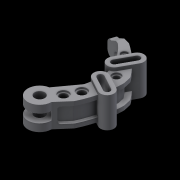
# Autodesk Inventor part: new clamp
Saved by Autodesk Inventor 2015 (Build 190159000, 159)
## iProperties
Created: 2014-10-18
Part Number: new clamp
Material: Generic
Document SubType Name: Modeling
Designer: Inventor
Mass: 7.61279 g
Surface Area: 66.4812 cm^2
Volume: 7.61279 cm^3
Density: 1 g/cm^3
Appearance: Default
RuleStatus: InUse
BeforeDocSave0: UpdateBoundingBox
CX: 35.89 mm
CY: 63.14 mm
CZ: 18.00 mm
Author: Inventor
Autodesk Inventor part; units mm, degrees
ref_plane "YZ Plane" through (0, 0, 0) normal (1, 0, 0) x (0, 1, 0)
ref_plane "XZ Plane" through (0, 0, 0) normal (0, 1, 0) x (-1, 0, 0)
ref_plane "XY Plane" through (0, 0, 0) normal (0, 0, 1) x (1, 0, 0)
sketch "Base" plane through (0, 0, 0) normal (0, 0, 1) x (1, 0, 0)
  circle A0 centre (0, 0) radius 26 construction
  line L0 (17.6916, -25.456) -> (27.5664, -11.8645) construction
  line L1 (27.5664, -11.8645) -> (28.9894, 8.4858) construction
  line L2 (28.9894, 8.4858) -> (16.9443, 25.688) construction
  line L3 (16.9443, 25.688) -> (5.3532, 28.7938) construction
  arc A1 (30.9898, -18.2111) -> (36.4924, 5.7494) centre (-19.9066, 6.0896) ccw
  line L4 (24.6916, -25.4563) -> (30.9898, -18.2111)
  arc A2 (35.4682, 10.4389) -> (17.4626, 27.6222) centre (-24.5964, -34.4748) ccw
  line L5 (35.4682, 10.4389) -> (36.4924, 5.7494)
  line L6 (17.4626, 27.6222) -> (5.8715, 30.728)
  line L7 (5.8715, 30.728) -> (4.9656, 27.3473)
  arc A3 (25.6196, 7.5403) -> (14.0958, 24.3807) centre (-10.6938, -4.9457) ccw
  line L8 (4.9656, 27.3473) -> (14.0958, 24.3807)
  circle A4 centre (17.6916, -25.456) radius 7
  line L9 (25.1124, -6.7357) -> (16.5261, -18.5537)
  circle A5 centre (29.4754, 20.4271) radius 1.75 construction
  line L10 (29.4754, 20.4271) -> (24.6884, 11.6473) construction
  circle A6 centre (24.6884, 11.6473) radius 1.75 construction
  circle A7 centre (29.4754, 20.4271) radius 4
  circle A8 centre (24.6884, 11.6473) radius 4
  circle A9 centre (28.0765, 0.1355) radius 1.75 construction
  line L11 (28.0765, 0.1355) -> (36.8564, -4.6514) construction
  circle A10 centre (36.8564, -4.6514) radius 1.75 construction
  circle A11 centre (36.8564, -4.6514) radius 4
  circle A12 centre (28.0765, 0.1355) radius 4
  line L12 (21.1765, 13.562) -> (25.9634, 22.3419)
  line L13 (28.2004, 9.7325) -> (32.9873, 18.5123)
  line L14 (29.9913, 3.6474) -> (38.7711, -1.1395)
  line L15 (26.1618, -3.3764) -> (34.9416, -8.1633)
  arc A13 (25.1124, -6.7357) -> (25.6196, 7.5403) centre (-5.602, 1.5026) ccw
  line L16 (0, 0) -> (26.0993, 7.6814) construction
  line L17 (16.9443, 25.688) -> (17.4626, 27.6222) construction
  line L18 (0, -47.5154) -> (0, 43.7686) construction
  line L19 (14.0958, 24.3807) -> (14.6134, 26.3126) construction
  line L20 (23.0874, 16.9148) -> (27.1832, 19.7827) construction
  line L21 (34.2322, -9.7203) -> (27.748, -9.2669) construction
  line L22 (24.6884, 11.6473) -> (28.0765, 0.1355) construction
  line L23 (-39.3713, 0) -> (54.2276, 0) construction
  line L24 (26.0993, 7.6814) -> (35.4682, 10.4389) construction
  dimension "d299" = 52
  dimension "d94" = 14
  dimension "d110" = 20.4
  dimension "d111" = 141
  dimension "d112" = 21
  dimension "d122" = 3.5
  dimension "d124" = 8
  dimension "d137" = 16.8
  dimension "d138" = 148
  dimension "d143" = 135
  dimension "d144" = 135
  dimension "d274" = 12
  dimension "d277" = 75
  dimension "d278" = 56.4
  dimension "d279" = 38.4
  dimension "d280" = 31.8
  dimension "d281" = 9.6
  dimension "d283" = 9.6
  dimension "d284" = 3.5
  dimension "d285" = 4.8
  dimension "d287" = 10
  dimension "d288" = 93
  dimension "d292" = 5
  dimension "d294" = 36
  dimension "d295" = 2
  dimension "d296" = 5
  dimension "d297" = 6.5
  dimension "d300" = 3
  dimension "d301" = 16.4
  dimension "d302" = 3.5
  dimension "d303" = 6.5
  dimension "d304" = 12
  dimension "d306" = 85.92
  dimension "d307" = 12
  dimension "d308" = 10
  dimension "d315" = 5
  dimension "d316" = 31
  dimension "d421" = 140
  constraints: 46 end point, 20 point on circle, 13 centre point, 9 coincident, 7 perpendicular, 7 tangent, 5 point on line, 4 equal radius, 4 parallel, 1 collinear, 4 other
  measures "d94" diameter of A4
  measures "d110" distance of L0.end L1.end
  measures "d111" angle of L1 L2
  measures "d112" distance of L1.end L2.end
  measures "d122" diameter of A5
  measures "d124" diameter of A7
  measures "d137" distance of L0.start L0.end
  measures "d138" angle of L0 L1
  measures "d143" angle of L10 L16
  measures "d144" angle of L11 L16
  measures "d274" distance of L2.end L3.end
  measures "d277" radius of A2
  measures "d278" radius of A1
  measures "d279" radius of A3
  measures "d280" radius of A13
  measures "d281" distance of L4.start L4.end
  measures "d283" distance of L7.end L8.end
  measures "d284" distance of L6.end L7.end
  measures "d285" distance of L5.start L5.end
  measures "d287" distance of L11.start L11.end
  measures "d288" angle of L7 L8
  measures "d292" angle of L4 L0
  measures "d294" angle of L18 L0
  measures "d295" distance of L8.end L19.end
  measures "d296" distance of L20.start L20.end
  measures "d297" distance of L21.start L21.end
  measures "d300" distance of L1.end L16.end
  measures "d301" angle of L16 L23
  measures "d302" distance of A3.start L1.end
  measures "d303" distance from line of L0 L4.end
  measures "d304" distance of L22.start L22.end
  measures "d306" angle of L24 L5
  measures "d307" vertical distance of L11.start L0.end
  measures "d308" distance from line of L5.start L22
  measures "d315" distance between parallel lines of L0 L9
  measures "d316" distance of point (0, 0) L0.start
  measures "d421" angle of L3 L2
extrude "BaseFeature" add sketch "Base" along normal blind 14
sketch "Rails" plane through (0, 0, 14) normal (0, 0, 1) x (1, 0, 0)
  arc A0 (21.1765, 13.562) -> (25.5499, 7.7411) centre (24.6884, 11.6473) ccw projected
  arc A1 (32.9873, 18.5123) -> (25.9634, 22.3419) centre (29.4754, 20.4271) ccw projected
  arc A2 (26.1269, 3.6282) -> (25.8502, -3.1877) centre (28.0765, 0.1355) ccw projected
  arc A3 (34.9416, -8.1633) -> (38.7711, -1.1395) centre (36.8564, -4.6514) ccw projected
  circle A4 centre (24.6884, 11.6473) radius 1.75
  circle A5 centre (29.4754, 20.4271) radius 1.75
  circle A6 centre (36.8564, -4.6514) radius 1.75
  circle A7 centre (28.0765, 0.1355) radius 1.75
  line L0 (27.9389, 21.2648) -> (23.152, 12.485)
  line L1 (26.2249, 10.8096) -> (31.0118, 19.5894)
  line L2 (28.9143, 1.672) -> (37.6941, -3.1149)
  line L3 (36.0187, -6.1879) -> (27.2388, -1.401)
  point P0 (25.6248, -3.3764)
  point P1 (34.4326, -8.1784)
  point P2 (29.3887, 7.0803)
  point P3 (21.8452, 13.2008)
  point P4 (25.5283, 6.9564)
  dimension "d148" = 3.5
  dimension "d149" = 3.5
  dimension "d150" = 3.5
  dimension "d151" = 3.5
  constraints: 8 end point, 8 point on circle, 7 tangent, 4 centre point, 4 coincident, 1 parallel, 3 other
  measures "d148" diameter of A4
  measures "d149" diameter of A5
  measures "d150" diameter of A6
  measures "d151" diameter of A7
extrude "RailsFeature" cut sketch "Rails" against normal through all
sketch "EndTaper" plane through (14.0958, 24.3807, 0) normal (-0.309017, -0.9510565, 0) x (0.9510565, -0.309017, 0)
  line L0 (-9.6, 0) -> (0, 0) projected
  line L1 (0, 0) -> (0, 14) projected
  line L2 (-9.6, 14) -> (0, 14) projected
  line L3 (-9.6, 0) -> (-9.6, 14) construction
  line L4 (0, 0) -> (0, 14) projected
  line L5 (-6.0622, 2.5) -> (-9.6, 2.5)
  line L6 (-9.6, 2.5) -> (-9.6, 11.5)
  line L7 (-9.6, 11.5) -> (-6.0622, 11.5)
  line L8 (0, 15) -> (-10.7832, 15)
  line L9 (-10.7832, 15) -> (-10.7832, -1)
  line L10 (-10.7832, -1) -> (0, -1)
  line L11 (0, -1) -> (-6.0622, 2.5)
  line L12 (-6.0622, 11.5) -> (0, 15)
  line L13 (0, -1) -> (0, 15) construction
  line L14 (-9.7832, 0) -> (-9.7832, 14) construction
  line L15 (-6.0622, 2.5) -> (-6.0622, 11.5) construction
  dimension "d154" = 9
  dimension "d155" = 2.5
  dimension "d163" = 1
  dimension "d164" = 1
  dimension "d165" = 1
  dimension "d166" = 120
  dimension "d199" = 14
  constraints: 20 end point, 3 vertical, 2 collinear, 2 parallel, 2 perpendicular, 1 horizontal
  measures "d154" distance between parallel lines of L7 L5
  measures "d155" distance between parallel lines of L2 L7
  measures "d163" distance between parallel lines of L9 L14
  measures "d164" distance between parallel lines of L10 L0
  measures "d165" distance between parallel lines of L8 L2
  measures "d166" angle of L11 L15
  measures "d199" distance of L0.start L2.start
extrude "EndTaperFeature" cut sketch "EndTaper" against normal through all contours L11 L10 L9 L8 L12 L7 L6 L5
fillet "EndTaperFilletFeature" radius 3 2 edges at (5.5071, 29.0139, 2.5) (5.5071, 29.0139, 11.5)
sketch "RailBordersFront" plane through (0, 0, 14) normal (0, 0, 1) x (1, 0, 0)
  circle A0 centre (29.4754, 20.4271) radius 4 construction
  line L0 (28.2004, 9.7325) -> (32.9873, 18.5123) construction
  line L1 (21.1765, 13.562) -> (25.9634, 22.3419) construction
  line L2 (26.2249, 10.8096) -> (31.0118, 19.5894) construction
  circle A1 centre (29.4754, 20.4271) radius 1.75 construction
  circle A2 centre (24.6884, 11.6473) radius 1.75 construction
  line L3 (27.9389, 21.2648) -> (23.152, 12.485) construction
  line L4 (29.9913, 3.6474) -> (38.7711, -1.1395) construction
  circle A3 centre (36.8564, -4.6514) radius 4 construction
  circle A4 centre (28.0765, 0.1355) radius 4 construction
  line L5 (26.1618, -3.3764) -> (34.9416, -8.1633) construction
  circle A5 centre (28.0765, 0.1355) radius 1.75 construction
  circle A6 centre (36.8564, -4.6514) radius 1.75 construction
  line L6 (37.6941, -3.1149) -> (28.9143, 1.672) construction
  line L7 (27.2388, -1.401) -> (36.0187, -6.1879) construction
  circle A7 centre (24.6884, 11.6473) radius 4 construction
  arc A8 (32.9873, 18.5123) -> (25.9634, 22.3419) centre (29.4754, 20.4271) ccw
  arc A9 (21.1765, 13.562) -> (28.2004, 9.7325) centre (24.6884, 11.6473) ccw
  arc A10 (29.9913, 3.6474) -> (26.1618, -3.3764) centre (28.0765, 0.1355) ccw
  arc A11 (34.9416, -8.1633) -> (38.7711, -1.1395) centre (36.8564, -4.6514) ccw
  arc A12 (34.9416, -8.1633) -> (38.7711, -1.1395) centre (36.8564, -4.6514) ccw projected
  line L8 (25.9634, 22.3419) -> (21.1765, 13.562)
  line L9 (32.9873, 18.5123) -> (28.2004, 9.7325)
  line L10 (29.9913, 3.6474) -> (38.7711, -1.1395)
  line L11 (26.1618, -3.3764) -> (34.9416, -8.1633)
  arc A13 (31.0118, 19.5894) -> (27.9389, 21.2648) centre (29.4754, 20.4271) ccw
  arc A14 (23.152, 12.485) -> (26.2249, 10.8096) centre (24.6884, 11.6473) ccw
  arc A15 (28.9143, 1.672) -> (27.2388, -1.401) centre (28.0765, 0.1355) ccw
  arc A16 (36.0187, -6.1879) -> (37.6941, -3.1149) centre (36.8564, -4.6514) ccw
  line L12 (27.9389, 21.2648) -> (23.152, 12.485)
  line L13 (31.0118, 19.5894) -> (26.2249, 10.8096)
  line L14 (27.2388, -1.401) -> (36.0187, -6.1879)
  line L15 (28.9143, 1.672) -> (37.6941, -3.1149)
  constraints: 28 point on circle, 19 end point, 9 concentric, 8 centre point, 8 coincident, 8 collinear, 1 point on line
extrude "RailBordersFrontFeature" add sketch "RailBordersFront" along normal blind 2
sketch "RailBordersBack" plane through (0, 0, 0) normal (0, 0, -1) x (-1, 0, 0)
  line L0 (-23.152, 12.485) -> (-27.9389, 21.2648) projected
  arc A0 (-27.9389, 21.2648) -> (-31.0118, 19.5894) centre (-29.4754, 20.4271) ccw projected
  line L1 (-31.0118, 19.5894) -> (-26.2249, 10.8096) projected
  arc A1 (-26.2249, 10.8096) -> (-23.152, 12.485) centre (-24.6884, 11.6473) ccw projected
  arc A2 (-28.2004, 9.7325) -> (-21.1765, 13.562) centre (-24.6884, 11.6473) ccw projected
  line L2 (-28.2004, 9.7325) -> (-32.9873, 18.5123) projected
  arc A3 (-25.9634, 22.3419) -> (-32.9873, 18.5123) centre (-29.4754, 20.4271) ccw projected
  line L3 (-25.9634, 22.3419) -> (-21.1765, 13.562) projected
  line L4 (-36.0187, -6.1879) -> (-27.2388, -1.401) projected
  arc A4 (-27.2388, -1.401) -> (-28.9143, 1.672) centre (-28.0765, 0.1355) ccw projected
  line L5 (-28.9143, 1.672) -> (-37.6941, -3.1149) projected
  arc A5 (-37.6941, -3.1149) -> (-36.0187, -6.1879) centre (-36.8564, -4.6514) ccw projected
  line L6 (-38.7711, -1.1395) -> (-29.9913, 3.6474) projected
  arc A6 (-26.1618, -3.3764) -> (-29.9913, 3.6474) centre (-28.0765, 0.1355) ccw projected
  line L7 (-26.1618, -3.3764) -> (-34.9416, -8.1633) projected
  arc A7 (-38.7711, -1.1395) -> (-34.9416, -8.1633) centre (-36.8564, -4.6514) ccw projected
extrude "RailBordersBackFeature" add sketch "RailBordersBack" along normal blind 2
sketch "Trench1" plane through (17.4626, 27.6222, 14) normal (0.258819, 0.9659258, 0) x (0.9659258, -0.258819, 0)
  ellipse E0 centre (-8.8125, 5.5) end of major axis (-11.8166, 5.5) minor radius 3 (-11.8166, 5.5) -> (-8.8125, 2.5) ccw projected
  line L0 (-8.8125, 2.5) -> (-8.2739, 2.5) projected
  line L1 (-8.2739, 2.5) -> (-3.9378, 0) projected
  line L2 (0, 0) -> (-3.9378, 0) projected
  line L3 (0, 14) -> (0, 0) projected
  line L4 (0, 14) -> (-3.9378, 14) projected
  line L5 (-3.9378, 14) -> (-8.2739, 11.5) projected
  line L6 (-8.2739, 11.5) -> (-8.8125, 11.5) projected
  ellipse E1 centre (-8.8125, 8.5) end of major axis (-11.8166, 8.5) minor radius 3 (-8.8125, 11.5) -> (-11.8166, 8.5) ccw projected
  line L7 (-11.8166, 8.5) -> (-11.8166, 5.5) projected
  line L8 (9.3229, 14) -> (9.3229, 0) projected
  line L9 (9.3229, 14) -> (0, 14) projected
  line L10 (0, 14) -> (0, 0) projected
  line L11 (9.3229, 0) -> (0, 0) projected
  line L12 (-9.8166, 5.5) -> (-9.8166, 8.5)
  line L13 (-8.8125, 9.5) -> (-7.7386, 9.5)
  line L14 (-7.7386, 9.5) -> (-3.4026, 12)
  line L15 (-3.4026, 12) -> (0, 12)
  line L16 (0, 2) -> (-3.4026, 2)
  line L17 (-3.4026, 2) -> (-7.7386, 4.5)
  line L18 (-7.7386, 4.5) -> (-8.8125, 4.5)
  line L19 (0, 2) -> (0, 12)
  line L20 (16.5436, 0) -> (16.5436, 14) projected
  line L21 (21.8395, 0) -> (16.5436, 0) projected
  line L22 (21.8395, 14) -> (21.8395, 0) projected
  line L23 (21.8395, 14) -> (16.5436, 14) projected
  spline S0 degree 5 poles (-8.8125, 4.5) (-9.1273, 4.4999) (-9.4422, 4.6225) (-9.6924, 4.87) (-9.8166, 5.1851) (-9.8166, 5.5) knots 0 0 0 0 0 0 1 1 1 1 1 1
  spline S1 degree 5 poles (-9.8166, 8.5) (-9.8166, 8.8149) (-9.6924, 9.13) (-9.4422, 9.3775) (-9.1273, 9.5001) (-8.8125, 9.5) knots 0 0 0 0 0 0 1 1 1 1 1 1
  dimension "d185" = 2
  dimension "d212" = 2
  constraints: 16 end point, 3 parallel, 1 collinear, 1 vertical, 12 other
  measures "d212" distance between parallel lines of L0 L18
extrude "Trench1Feature" cut sketch "Trench1" against normal blind 2 contours L16 L17 L18 S0 L12 S1 L13 L14 L15 L3
ref_plane "MiddlePlane" through (0, 0, 7) normal (0, 0, 1) x (1, 0, 0)
sketch "BottomCut" plane through (0, 0, 7) normal (0, 0, 1) x (1, 0, 0)
  arc A0 (16.5261, -18.5537) -> (24.6916, -25.4563) centre (17.6916, -25.456) ccw projected
  circle A1 centre (17.6916, -25.456) radius 7
  constraints: 1 coincident, 3 other
extrude "BottomCutFeature" cut sketch "BottomCut" along normal mid plane 5
sketch "Trench2" plane through (0, 0, 7) normal (0, 0, 1) x (1, 0, 0)
  arc A0 (35.4682, 10.4389) -> (31.3384, 15.4881) centre (-24.5964, -34.4748) ccw projected
  line L0 (36.4924, 5.7494) -> (35.4682, 10.4389) projected
  arc A1 (36.192, 0.2667) -> (36.4924, 5.7494) centre (-19.9066, 6.0896) ccw projected
  arc A2 (32.6776, 9.1565) -> (29.8097, 12.6842) centre (-24.5964, -34.4748) ccw
  line L1 (32.6776, 9.1565) -> (33.4895, 5.4391)
  arc A3 (33.3233, 1.8308) -> (33.4895, 5.4391) centre (-19.9066, 6.0896) ccw
  line L2 (28.2004, 9.7325) -> (32.9873, 18.5123) projected
  line L3 (38.7711, -1.1395) -> (29.9913, 3.6474) projected
  point P0 (-20.854, 3.4342)
  point P1 (-22.9622, -38.0663)
  dimension "d312" = 3
  dimension "d313" = 3
  dimension "d317" = 3
  constraints: 4 point on circle, 2 centre point, 2 end point, 2 point on line
  measures "d312" distance between parallel lines of L1 L0
  measures "d313" radial gap between concentric circles of A1 A3
  measures "d317" radial gap between concentric circles of A0 A2
extrude "Trench2Feature" cut sketch "Trench2" along normal mid plane 9
sketch "Trench3" plane through (0, 0, 7) normal (0, 0, 1) x (1, 0, 0)
  line L0 (25.9634, 22.3419) -> (21.1765, 13.562) construction
  arc A0 (25.4446, 21.3902) -> (17.4626, 27.6222) centre (-24.5964, -34.4748) ccw construction
  line L1 (17.4626, 27.6222) -> (16.945, 25.6903) construction
  arc A1 (25.4446, 21.3902) -> (17.4626, 27.6222) centre (-24.5964, -34.4748) ccw
  line L2 (17.4626, 27.6222) -> (16.945, 25.6903)
  arc A2 (24.516, 19.687) -> (16.945, 25.6903) centre (-24.5964, -34.4748) ccw
  line L3 (25.4446, 21.3902) -> (24.516, 19.687)
  point P0 (-19.1624, -33.4404)
  constraints: 4 end point, 4 point on circle, 2 centre point, 2 collinear
extrude "Trench3Feature" cut sketch "Trench3" along normal mid plane 10
sketch "Trench4" plane through (0, 0, 7) normal (0, 0, 1) x (1, 0, 0)
  arc A0 (30.9898, -18.2111) -> (36.4924, 5.7494) centre (-19.9066, 6.0896) ccw projected
  line L0 (24.6916, -25.4563) -> (30.9898, -18.2111) projected
  arc A1 (29.3004, -17.106) -> (32.8848, -7.0419) centre (-19.9066, 6.0896) ccw
  line L1 (29.3004, -17.106) -> (24.7619, -22.327)
  line L2 (32.8848, -7.0419) -> (39.0853, -10.4225)
  line L3 (39.0853, -10.4225) -> (27.026, -24.2951)
  line L4 (27.026, -24.2951) -> (24.7619, -22.327)
  arc A2 (24.6916, -25.4563) -> (16.5261, -18.5537) centre (17.6916, -25.456) ccw projected
  line L5 (26.1618, -3.3764) -> (34.9416, -8.1633) projected
  dimension "d232" = 2
  dimension "d233" = 3
  constraints: 8 end point, 2 perpendicular, 2 point on circle, 1 centre point, 1 collinear, 1 tangent, 1 other
  measures "d232" radial gap between concentric circles of A0 A1
  measures "d233" distance of L3.end L1.end
extrude "Trench4Feature" cut sketch "Trench4" along normal mid plane 9
fillet "AngleFilletsFeature" radius 3 11 edges at (17.4626, 27.6222, 1) (17.4626, 27.6222, 13) (35.4682, 10.4389, 1.25) (35.4682, 10.4389, 12.75) (36.4924, 5.7494, 12.75) (36.4924, 5.7494, 1.25) (29.3004, -17.106, 7) (30.9898, -18.2111, 1.25) (30.9898, -18.2111, 12.75) (14.0958, 24.3807, 7) (25.1124, -6.7357, 7)
fillet "TrenchInsideFilletsFeature" radius 1.5 2 edges at (25.5166, -22.983, 2.5) (25.5166, -22.983, 11.5)
sketch "MountHole" plane through (0, 0, 14) normal (0, 0, 1) x (1, 0, 0)
  arc A0 (16.5261, -18.5537) -> (24.6916, -25.4563) centre (17.6916, -25.456) ccw projected
hole "MountHoleFeature" at (17.6916, -25.456, 14) direction (0, 0, -1) diameter 6 end through all
sketch "BaseHoles" plane through (0, 0, 14) normal (0, 0, 1) x (1, 0, 0)
  circle A0 centre (30.5552, 7.1577) radius 1.75
  circle A1 centre (24.2522, -17.9089) radius 2.25
  circle A2 centre (28.1307, -10.9119) radius 2.25
  circle A3 centre (21.6719, 20.7378) radius 1.25
  line L0 (24.7774, -7.1967) -> (16.5261, -18.5537) projected
  line L1 (24.6916, -25.4563) -> (30.7186, -18.5231) projected
  line L2 (26.1618, -3.3764) -> (34.9416, -8.1633) projected
  circle A4 centre (17.6916, -25.456) radius 3 projected
  line L3 (17.6916, -25.456) -> (24.2522, -17.9089) construction
  line L4 (24.2522, -17.9089) -> (28.1307, -10.9119) construction
  line L5 (28.2004, 9.7325) -> (32.9873, 18.5123) projected
  line L6 (36.4204, 6.0792) -> (35.6085, 9.7966) construction
  line L7 (25.9634, 22.3419) -> (21.1765, 13.562) construction
  line L8 (21.6719, 20.7378) -> (24.3059, 19.3017) construction
  circle A5 centre (21.6719, 20.7378) radius 2
  arc A6 (22.0356, 15.1378) -> (14.5707, 23.9726) centre (-10.6938, -4.9457) ccw projected
  dimension "d341" = 3.5
  dimension "d342" = 4.5
  dimension "d343" = 4.5
  dimension "d344" = 2.5
  dimension "d345" = 168
  dimension "d346" = 8
  dimension "d347" = 10
  dimension "d349" = 3
  dimension "d388" = 4
  dimension "d423" = 5.6
  dimension "d428" = 5.5
  dimension "d429" = 3.3
  constraints: 6 end point, 5 centre point, 1 coincident, 1 parallel, 1 perpendicular, 1 point on line
  measures "d341" diameter of A0
  measures "d342" diameter of A1
  measures "d343" diameter of A2
  measures "d344" diameter of A3
  measures "d345" angle of L4 L3
  measures "d346" distance of L3.end L4.end
  measures "d347" distance of L3.start L3.end
  measures "d349" distance of L8.start L8.end
  measures "d388" diameter of A5
  measures "d423" vertical distance of A6.start L8.start
  measures "d428" distance from line of L6 A0.centre
  measures "d429" distance from line of L5 A0.centre
extrude "BaseHole1ReinforceFeature" add sketch "BaseHoles" against normal through all contours A5
hole "BaseHole1Feature" at (21.6719, 20.7378, 14) direction (0, 0, -1) diameter 2.5 end through all counterbore diameter 4 counterbore depth 1
hole "BaseHole2Feature" at (30.5552, 7.1577, 14) direction (0, 0, -1) diameter 3.5 end through all counterbore diameter 5 counterbore depth 1
hole "BaseHole3Feature" at (28.1307, -10.9119, 14) direction (0, 0, -1) diameter 4.5 end through all counterbore diameter 6 counterbore depth 1
hole "BaseHole4Feature" at (24.2522, -17.9089, 14) direction (0, 0, -1) diameter 4.5 end through all counterbore diameter 6 counterbore depth 1
sketch "EndHole" plane through (16.945, 25.6903, 14) normal (0.258819, 0.9659258, 0) x (0.9659258, -0.258819, 0)
  circle A0 centre (-3.8166, 7) radius 1.75
  line L0 (-9.8166, 5.5) -> (-9.8166, 8.5) projected
  line L1 (0.4915, 2) -> (9.3229, 2) construction
  line L2 (9.3229, 12) -> (0.4915, 12) construction
  dimension "d378" = 3.5
  dimension "d425" = 5
  dimension "d426" = 5
  dimension "d427" = 6
  constraints: 1 centre point, 1 coincident
  measures "d378" diameter of A0
  measures "d425" distance from line of point (-3.817, 7) L1
  measures "d426" distance from line of L2 point (-3.817, 7)
  measures "d427" distance from line of L0 point (-3.817, 7)
hole "EndHoleFeature" at (13.2584, 26.6782, 7) direction (-0.258819, -0.9659258, 0) diameter 3.5 end through all
sketch "BaseHolesBackDetail" plane through (0, 0, 0) normal (0, 0, -1) x (-1, 0, 0)
  circle A0 centre (-21.6719, 20.7378) radius 2 projected
  circle A1 centre (-21.6719, 20.7378) radius 2 projected
  circle A2 centre (-21.6719, 20.7378) radius 1.25 projected
  circle A3 centre (-30.5552, 7.1577) radius 2.5 projected
  circle A4 centre (-30.5552, 7.1577) radius 1.75 projected
  circle A5 centre (-28.1307, -10.9119) radius 3 projected
  circle A6 centre (-28.1307, -10.9119) radius 2.25 projected
  circle A7 centre (-24.2522, -17.9089) radius 3 projected
  circle A8 centre (-24.2522, -17.9089) radius 2.25 projected
extrude "BaseHolesDetailFeature" cut sketch "BaseHolesBackDetail" against normal blind 1
equation "\"d155\" = -0.5 * d154 + 0.5 * d199"
